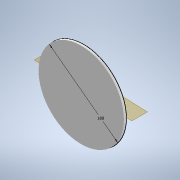
# Autodesk Inventor part: plošča za vrtenje
Saved by Autodesk Inventor 2022 (Build 260153000, 153)
## iProperties
Created: 2022-03-14
Part Number: plošča za vrtenje
Material: Generic
Document SubType Name: Modeling
Designer: simon
Density: 1 g/cm^3
Appearance: Default
Author: simon
Autodesk Inventor part; units mm, degrees
ref_plane "YZ Plane" through (0, 0, 0) normal (1, 0, 0) x (0, 1, 0)
ref_plane "XZ Plane" through (0, 0, 0) normal (0, 1, 0) x (-1, 0, 0)
ref_plane "XY Plane" through (0, 0, 0) normal (0, 0, 1) x (1, 0, 0)
sketch "Sketch1" plane through (0, 0, 0) normal (0, 0, 1) x (1, 0, 0)
  circle A0 centre (0, 0) radius 6.5
  dimension "d0" = 13
  constraints: 1 centre point, 1 coincident
  measures "d0" diameter of A0
extrude "Extrusion1" add sketch "Sketch1" along normal blind 30
sketch "Sketch3" plane through (0, 0, 30) normal (0, 0, 1) x (1, 0, 0)
  circle A0 centre (0, 0) radius 90
  dimension "d3" = 180
  constraints: 1 centre point, 1 coincident
  measures "d3" diameter of A0
sketch "Sketch4" plane through (0, 0, 0) normal (0, 0, -1) x (-1, 0, 0)
  circle A0 centre (0, 0) radius 2
  dimension "d4" = 4
  constraints: 1 centre point, 1 coincident
  measures "d4" diameter of A0
extrude "Extrusion2" cut sketch "Sketch4" against normal blind 20
ref_plane "Work Plane2" through (0.2663, 6.4945, 0) normal (0.041, 0.9992, 0) x (-0.9992, 0.041, 0)
ref_plane "Work Plane1" through (-27.6829, 45.9903, 12) normal (0.041, 0.9992, 0) x (-0.9992, 0.041, 0)
ref_plane "Work Plane4" through (0.2663, 6.4945, 0) normal (0.041, 0.9992, 0) x (-0.9992, 0.041, 0)
ref_plane "Work Plane3" through (19.1559, -19.777, -43.8) normal (0.041, 0.9992, 0) x (-0.9992, 0.041, 0)
sketch "Sketch5" plane through (0.2663, 6.4945, 0) normal (0.041, 0.9992, 0) x (-0.9992, 0.041, 0)
  line L0 (0, 0) -> (0, 20)
  line L1 (0, 20) -> (0, 5)
  line L2 (0, 5) -> (0, 10)
  circle A0 centre (0, 10) radius 1.2
  circle A1 centre (0, 5) radius 1.2
  dimension "d7" = 20
  dimension "d8" = 15
  dimension "d9" = 5
  dimension "d10" = 2.4
  constraints: 6 end point, 2 centre point, 2 coincident, 2 point on line, 1 vertical
  measures "d7" distance of L0.start L0.end
  measures "d8" distance of L0.end L1.end
  measures "d9" distance of L1.end L2.end
  measures "d10" diameter of A0
extrude "Extrusion3" cut sketch "Sketch5" against normal blind 20
sketch "Sketch6" plane through (0, 0, 30) normal (0, 0, 1) x (1, 0, 0)
  circle A0 centre (0, 0) radius 90
  dimension "d13" = 180
  constraints: 1 centre point, 1 coincident
  measures "d13" diameter of A0
extrude "Extrusion4" add sketch "Sketch6" along normal blind 5
body "Solid1"
